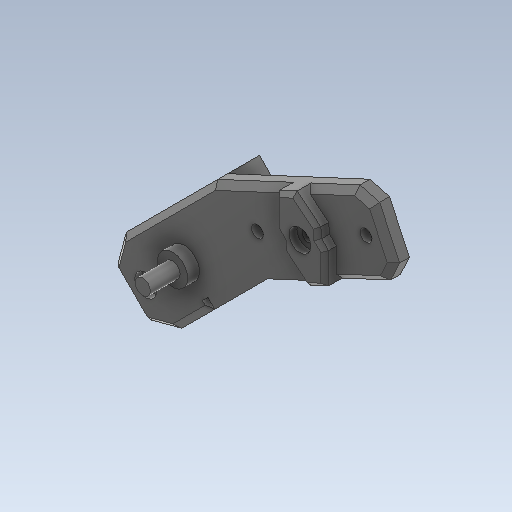
# Autodesk Inventor part: Tibia2Top
Saved by Autodesk Inventor 2020 (Build 240168000, 168)
## iProperties
Created: 2020-09-11
Part Number: Tibia2Top
Material: Generic
Document SubType Name: Modeling
Designer: Turing
Density: 1 g/cm^3
Appearance: Smooth - Black
Mass: 12.5949 g
Surface Area: 55.3576 cm^2
Volume: 12.5949 cm^3
Author: Turing
Autodesk Inventor part; units mm, degrees
ref_plane "YZ Plane" through (0, 0, 0) normal (1, 0, 0) x (0, 1, 0)
ref_plane "XZ Plane" through (0, 0, 0) normal (0, 1, 0) x (-1, 0, 0)
ref_plane "XY Plane" through (0, 0, 0) normal (0, 0, 1) x (1, 0, 0)
sketch "Sketch1" plane through (0, 0, 0) normal (0, 0, 1) x (1, 0, 0)
  circle A0 centre (158.1587, -44.9831) radius 1.5
  circle A1 centre (158.1574, -44.9818) radius 3.6
  line L0 (162.4482, -44.088) -> (170.4914, -34.8578)
  line L1 (167.6018, -32.12) -> (158.8186, -40.6491)
  circle A2 centre (168.8869, -33.6576) radius 1.9999
  line L2 (161.7538, -44.8209) -> (162.4482, -44.088)
  line L3 (158.1242, -41.382) -> (158.8186, -40.6491)
  line L4 (158.1574, -44.9818) -> (168.1574, -44.9818) construction
  line L5 (165.2285, -52.0529) -> (179.3706, -37.9108)
  line L6 (158.1574, -44.9818) -> (168.1574, -44.9818) construction
  line L7 (158.1574, -44.9818) -> (151.0863, -37.9108)
  line L8 (151.0863, -37.9108) -> (165.2285, -23.7686)
  line L9 (165.2285, -23.7686) -> (201.4808, -6.8639)
  line L10 (179.3706, -37.9108) -> (206.5598, -25.2322)
  line L11 (151.0863, -37.9108) -> (141.894, -47.1032)
  line L12 (165.2285, -52.0529) -> (156.0361, -61.2453)
  line L13 (148.3087, -63.3158) -> (156.0361, -61.2453)
  line L14 (141.894, -47.1032) -> (139.8234, -54.8306)
  line L15 (148.3087, -63.3158) -> (139.8234, -54.8306)
  line L16 (209.2788, -23.9644) -> (206.5598, -25.2322)
  line L17 (201.4808, -6.8639) -> (206.4848, -8.2047)
  line L18 (206.4848, -8.2047) -> (211.5562, -19.0804)
  line L19 (211.5562, -19.0804) -> (209.2788, -23.9644)
  point P0 (0, 0)
  point P1 (167.4372, -32.2799)
  point P2 (167.5524, -32.168)
  point P3 (170.4476, -34.9082)
  point P4 (170.3392, -35.0325)
extrude "Extrusion2" add sketch "Sketch1" along normal mid plane 7.5 contours A0 | A1 | A1 L3 L1 A2 L0 L2 | A2 | L12 L13 L15 L14 L11 L8 L9 L17 L18 L19 L16 L10 L5
sketch "Sketch9" plane through (0, 0, 3.75) normal (0, 0, 1) x (1, 0, 0)
  line L0 (156.0361, -61.2453) -> (179.3706, -37.9108) projected
  line L1 (179.3706, -37.9108) -> (209.2788, -23.9644) projected
  line L2 (201.4808, -6.8639) -> (165.2285, -23.7686) projected
  line L3 (165.2285, -23.7686) -> (141.894, -47.1032) projected
  line L4 (141.894, -47.1032) -> (139.8234, -54.8306) projected
  line L5 (139.8234, -54.8306) -> (148.3087, -63.3158) projected
  line L6 (148.3087, -63.3158) -> (156.0361, -61.2453) projected
  line L7 (209.2788, -23.9644) -> (211.5562, -19.0804) projected
  line L8 (211.5562, -19.0804) -> (206.4848, -8.2047) projected
  line L9 (206.4848, -8.2047) -> (201.4808, -6.8639) projected
  point P0 (0, 0)
extrude "Extrusion10" add sketch "Sketch9" along normal blind 5
sketch "Sketch10" plane through (0, 0, 8.75) normal (0, 0, 1) x (1, 0, 0)
  circle A0 centre (158.1587, -44.9831) radius 1.5 projected
  circle A1 centre (158.1587, -44.9831) radius 3.88
  point P0 (0, 0)
  dimension "d155" = 2.38
  constraints: 1 centre point
  measures "d155" radial gap between concentric circles of A0 A1
extrude "Extrusion11" add sketch "Sketch10" along normal blind 3 contours A0 | A1
sketch "Sketch11" plane through (158.1587, -44.9831, 11.75) normal (0, 0, 1) x (1, 0, 0)
  circle A0 centre (0, 0) radius 1.65 projected
  circle A1 centre (0, 0) radius 1.55
  point P0 (-158.1587, 44.9831)
  dimension "d158" = 0.1
  constraints: 1 centre point
  measures "d158" radial gap between concentric circles of A0 A1
extrude "Extrusion12" add sketch "Sketch11" along normal blind 7.6 contours A1
sketch "Sketch15" plane through (0, 0, -3.75) normal (0, 0, -1) x (-1, 0, 0)
  line L0 (-165.2285, -23.7686) -> (-201.4808, -6.8639) projected
  line L1 (-201.4808, -6.8639) -> (-206.4848, -8.2047) projected
  line L2 (-206.4848, -8.2047) -> (-211.5562, -19.0804) projected
  line L3 (-211.5562, -19.0804) -> (-209.2788, -23.9644) projected
  line L4 (-209.2788, -23.9644) -> (-179.3706, -37.9108) projected
  line L5 (-179.3706, -37.9108) -> (-156.0361, -61.2453) projected
  line L6 (-156.0361, -61.2453) -> (-148.3087, -63.3158) projected
  line L7 (-148.3087, -63.3158) -> (-139.8234, -54.8306) projected
  line L8 (-139.8234, -54.8306) -> (-141.894, -47.1032) projected
  line L9 (-141.894, -47.1032) -> (-165.2285, -23.7686) projected
  point P0 (0, 0)
extrude "Extrusion15" cut sketch "Sketch15" against normal blind 0.4
sketch "Sketch25" plane through (0, 0, -3.35) normal (0, 0, -1) x (-1, 0, 0)
  line L0 (-156.0361, -61.2453) -> (-179.3706, -37.9108) projected
  line L1 (-148.3087, -63.3158) -> (-156.0361, -61.2453) projected
  line L2 (-139.8234, -54.8306) -> (-148.3087, -63.3158) projected
  line L3 (-141.894, -47.1032) -> (-139.8234, -54.8306) projected
  line L4 (-165.2285, -23.7686) -> (-141.894, -47.1032) projected
  line L5 (-201.4808, -6.8639) -> (-165.2285, -23.7686) projected
  line L6 (-206.4848, -8.2047) -> (-201.4808, -6.8639) projected
  line L7 (-211.5562, -19.0804) -> (-206.4848, -8.2047) projected
  line L8 (-209.2788, -23.9644) -> (-211.5562, -19.0804) projected
  line L9 (-179.3706, -37.9108) -> (-209.2788, -23.9644) projected
  line L10 (-165.2285, -23.7686) -> (-179.3706, -37.9108)
  point P0 (0, 0)
  constraints: 2 end point
extrude "Extrusion23" cut sketch "Sketch25" against normal blind 8.1 contours L9 L8 L7 L6 L5 L10
sketch "Sketch26" plane through (0, 0, 4.75) normal (0, 0, -1) x (-1, 0, 0)
  line L0 (-201.4808, -6.8639) -> (-165.2285, -23.7686) projected
  line L1 (-206.4848, -8.2047) -> (-201.4808, -6.8639) projected
  line L2 (-211.5562, -19.0804) -> (-206.4848, -8.2047) projected
  line L3 (-209.2788, -23.9644) -> (-211.5562, -19.0804) projected
  line L4 (-179.3706, -37.9108) -> (-209.2788, -23.9644) projected
  line L5 (-165.2285, -23.7686) -> (-179.3706, -37.9108) projected
  line L6 (-209.0205, -13.6426) -> (-172.2995, -30.8397)
  line L7 (-172.2995, -30.8397) -> (-176.8276, -28.7191)
  circle A0 centre (-176.8276, -28.7191) radius 1.55
  line L8 (-209.0205, -13.6426) -> (-204.4924, -15.7631)
  circle A1 centre (-204.4924, -15.7631) radius 1.55
  line L9 (-190.66, -22.2411) -> (-190.6604, -22.242)
  circle A2 centre (-190.6604, -22.242) radius 1.5
  point P0 (0, 0)
  dimension "d262" = 5
  dimension "d263" = 3.1
  dimension "d264" = 5
  dimension "d265" = 3.1
  dimension "d270" = 90
  dimension "d271" = 0.001
  dimension "d272" = 3
  constraints: 8 end point, 3 centre point, 3 coincident, 3 midpoint, 2 point on line
  measures "d262" distance of L6.end L7.end
  measures "d263" diameter of A0
  measures "d264" distance of L6.start L8.end
  measures "d265" diameter of A1
  measures "d270" angle of L6 L9
  measures "d271" distance of L9.start L9.end
  measures "d272" diameter of A2
extrude "Extrusion24" cut sketch "Sketch26" against normal up to surface (4 mm away) contours A0 L6 | L6 A0 | A1 L6 | L6 A1 | A2 L6 | L6 A2
sketch "Sketch27" plane through (0, 0, -3.35) normal (0, 0, -1) x (-1, 0, 0)
  line L0 (-165.2285, -23.7686) -> (-179.3706, -37.9108) projected
  line L1 (-156.0361, -61.2453) -> (-179.3706, -37.9108) projected
  line L2 (-148.3087, -63.3158) -> (-156.0361, -61.2453) projected
  line L3 (-139.8234, -54.8306) -> (-148.3087, -63.3158) projected
  line L4 (-141.894, -47.1032) -> (-139.8234, -54.8306) projected
  line L5 (-165.2285, -23.7686) -> (-141.894, -47.1032) projected
  line L6 (-144.066, -59.0732) -> (-148.3087, -54.8306)
  circle A0 centre (-148.3087, -54.8306) radius 1.5
  point P0 (0, 0)
  dimension "d273" = 6
  dimension "d274" = 90
  dimension "d275" = 3
  constraints: 2 end point, 1 centre point, 1 coincident, 1 midpoint
  measures "d273" distance of L6.start L6.end
  measures "d274" angle of L6 L3
  measures "d275" diameter of A0
extrude "Extrusion25" cut sketch "Sketch27" against normal up to surface (12.1 mm away) contours A0
sketch "Sketch29" plane through (0, 0, 8.75) normal (0, 0, 1) x (1, 0, 0)
  circle A0 centre (148.3087, -54.8306) radius 1.5 projected
  circle A1 centre (204.4924, -15.7631) radius 1.55 projected
  circle A2 centre (190.6604, -22.242) radius 1.5 projected
  circle A3 centre (176.8276, -28.7191) radius 1.55 projected
  circle A4 centre (158.1587, -44.9831) radius 3.88 projected
  line L0 (211.5562, -19.0804) -> (206.4848, -8.2047) projected
  line L1 (206.4848, -8.2047) -> (201.4808, -6.8639) projected
  line L2 (201.4808, -6.8639) -> (165.2285, -23.7686) projected
  line L3 (165.2285, -23.7686) -> (141.894, -47.1032) projected
  line L4 (141.894, -47.1032) -> (139.8234, -54.8306) projected
  line L5 (139.8234, -54.8306) -> (148.3087, -63.3158) projected
  line L6 (148.3087, -63.3158) -> (156.0361, -61.2453) projected
  line L7 (156.0361, -61.2453) -> (179.3706, -37.9108) projected
  line L8 (179.3706, -37.9108) -> (209.2788, -23.9644) projected
  line L9 (209.2788, -23.9644) -> (211.5562, -19.0804) projected
  circle A5 centre (148.3087, -54.8306) radius 2.8
  point P0 (0, 0)
  dimension "d278" = 5.6
  constraints: 1 centre point, 1 coincident
  measures "d278" diameter of A5
extrude "Extrusion26" cut sketch "Sketch29" against normal blind 2 contours A0 | A5
sketch "Sketch30" plane through (0, 0, 8.75) normal (0, 0, 1) x (1, 0, 0)
  circle A0 centre (148.3087, -54.8306) radius 2.8 projected
  circle A1 centre (204.4924, -15.7631) radius 1.55 projected
  circle A2 centre (190.6604, -22.242) radius 1.5 projected
  circle A3 centre (176.8276, -28.7191) radius 1.55 projected
  circle A4 centre (158.1587, -44.9831) radius 3.88 projected
  line L0 (139.8234, -54.8306) -> (148.3087, -63.3158) projected
  line L1 (148.3087, -63.3158) -> (156.0361, -61.2453) projected
  line L2 (156.0361, -61.2453) -> (179.3706, -37.9108) projected
  line L3 (179.3706, -37.9108) -> (209.2788, -23.9644) projected
  line L4 (209.2788, -23.9644) -> (211.5562, -19.0804) projected
  line L5 (211.5562, -19.0804) -> (206.4848, -8.2047) projected
  line L6 (206.4848, -8.2047) -> (201.4808, -6.8639) projected
  line L7 (201.4808, -6.8639) -> (165.2285, -23.7686) projected
  line L8 (165.2285, -23.7686) -> (141.894, -47.1032) projected
  line L9 (141.894, -47.1032) -> (139.8234, -54.8306) projected
  line L10 (190.6604, -22.242) -> (194.6455, -30.788)
  line L11 (190.6604, -22.242) -> (186.7029, -13.755)
  line L12 (190.6604, -22.242) -> (195.192, -20.1289)
  line L13 (190.6604, -22.242) -> (186.1289, -24.3551)
  line L14 (186.1289, -24.3551) -> (184.3611, -22.5874)
  line L15 (186.1289, -24.3551) -> (186.3468, -26.8456)
  line L16 (195.192, -20.1289) -> (194.9741, -17.6385)
  line L17 (195.192, -20.1289) -> (196.9597, -21.8967)
  line L18 (194.6455, -30.788) -> (192.3797, -31.8445)
  line L19 (194.6455, -30.788) -> (196.9112, -29.7314)
  line L20 (186.7029, -13.755) -> (184.4371, -14.8115)
  line L21 (186.7029, -13.755) -> (188.9686, -12.6984)
  line L22 (192.3797, -31.8445) -> (186.3468, -26.8456)
  line L23 (196.9112, -29.7314) -> (196.9597, -21.8967)
  line L24 (194.9741, -17.6385) -> (188.9686, -12.6984)
  line L25 (184.3611, -22.5874) -> (184.4371, -14.8115)
  point P0 (0, 0)
  dimension "d281" = 90
  dimension "d282" = 90
  dimension "d283" = 90
  dimension "d284" = 90
  dimension "d285" = 5
  dimension "d286" = 5
  dimension "d287" = 2.5
  dimension "d288" = 2.5
  dimension "d289" = 2.5
  dimension "d291" = 110
  dimension "d292" = 110
  dimension "d293" = 110
  dimension "d295" = 110
  dimension "d296" = 2.5
  dimension "d297" = 2.5
  dimension "d298" = 2.5
  dimension "d299" = 2.5
  dimension "d300" = 2.5
  constraints: 32 end point, 6 point on line
  measures "d281" angle of L11 L7
  measures "d282" angle of L3 L10
  measures "d283" angle of L10 L13
  measures "d284" angle of L10 L12
  measures "d285" distance of L10.start L13.end
  measures "d286" distance of L10.start L12.end
  measures "d287" distance of L13.end L14.end
  measures "d288" distance of L13.end L15.end
  measures "d289" distance of L12.end L16.end
  measures "d291" angle of L15 L13
  measures "d292" angle of L13 L14
  measures "d293" angle of L16 L12
  measures "d295" angle of L17 L12
  measures "d296" distance of L12.end L17.end
  measures "d297" distance of L10.end L18.end
  measures "d298" distance of L19.end L10.end
  measures "d299" distance of L11.end L20.end
  measures "d300" distance of L11.end L21.end
extrude "Extrusion27" add sketch "Sketch30" along normal blind 3 contours A2 L12 L17 L23 L3 L10 | A2 L11 L7 L24 L16 L12 | L10 L3 L22 L15 L13 A2 | A2 L13 L14 L25 L7 L11
sketch "Sketch31" plane through (0, 0, 11.75) normal (0, 0, 1) x (1, 0, 0)
  line L0 (195.192, -20.1289) -> (194.9741, -17.6385) projected
  line L1 (194.9741, -17.6385) -> (188.9686, -12.6984) projected
  line L2 (188.9686, -12.6984) -> (184.4371, -14.8115) projected
  line L3 (184.4371, -14.8115) -> (184.3611, -22.5874) projected
  line L4 (184.3611, -22.5874) -> (186.1289, -24.3551) projected
  line L5 (186.1289, -24.3551) -> (186.3468, -26.8456) projected
  line L6 (186.3468, -26.8456) -> (192.3797, -31.8445) projected
  line L7 (192.3797, -31.8445) -> (196.9112, -29.7314) projected
  line L8 (196.9112, -29.7314) -> (196.9597, -21.8967) projected
  line L9 (196.9597, -21.8967) -> (195.192, -20.1289) projected
  circle A0 centre (190.6604, -22.242) radius 1.5 projected
  circle A1 centre (190.6604, -22.242) radius 2.8
  point P0 (0, 0)
  dimension "d307" = 5.6
  constraints: 1 centre point, 1 coincident
  measures "d307" diameter of A1
extrude "Extrusion28" cut sketch "Sketch31" against normal blind 2 contours A0 | A1
sketch "Sketch32" plane through (209.2788, -23.9644, 4.75) normal (0.4226183, -0.9063078, 0) x (0.9063078, 0.4226183, 0)
  line L0 (-33, 0) -> (0, 0) projected
  line L1 (0, 0) -> (0, 4) projected
  line L2 (-13.6461, 4) -> (0, 4) projected
  line L3 (-13.6461, 4) -> (-13.6461, 7) projected
  line L4 (-18.6461, 7) -> (-13.6461, 7) projected
  line L5 (-18.6461, 4) -> (-18.6461, 7) projected
  line L6 (-33, 4) -> (-18.6461, 4) projected
  line L7 (-33, 0) -> (-33, 4) projected
  line L8 (-16.1461, 7) -> (-16.1461, 2)
  line L9 (-16.1461, 2) -> (-33, 2)
  line L10 (-16.1461, 2) -> (-15.1461, 2)
  line L11 (-15.1461, 2) -> (-15.1461, 0)
  line L12 (-15.1461, 2) -> (-15.1461, 3)
  line L13 (-16.1461, 2) -> (-17.1461, 2)
  line L14 (-17.1461, 2) -> (-17.1461, 0)
  line L15 (-17.1461, 2) -> (-17.1461, 1)
  line L16 (-17.1461, 1) -> (-33, 1)
  line L17 (-15.1461, 3) -> (-33, 3)
  point P0 (-179.5432, -4.75)
  dimension "d310" = 90
  dimension "d311" = 1
  dimension "d312" = 1
  dimension "d313" = 1
  dimension "d314" = 1
  constraints: 20 end point, 6 point on line, 3 midpoint, 3 perpendicular, 2 vertical, 1 parallel
  measures "d310" angle of L8 L9
  measures "d311" distance of L8.end L10.end
  measures "d312" distance of L10.end L12.end
  measures "d313" distance of L8.end L13.end
  measures "d314" distance of L13.end L15.end
extrude "Extrusion29" cut sketch "Sketch32" against normal blind 2.5 contours L14 L9 L10 L11 L0 | L7 L9 L14 L16 | L7 L17 L8 L9 | L10 L8 L17 L12
sketch "Sketch34" plane through (156.0361, -61.2453, 8.75) normal (0.7071068, -0.7071068, 0) x (-0.7071068, -0.7071068, 0)
  line L0 (0, 12.1) -> (-33, 12.1) projected
  line L1 (-33, 12.1) -> (-33, 4) projected
  line L2 (-33, 4) -> (-33, 3) projected
  line L3 (-33, 3) -> (-33, 1) projected
  line L4 (-33, 1) -> (-33, 0) projected
  line L5 (0, 0) -> (-33, 0) projected
  line L6 (0, 12.1) -> (0, 0) projected
  line L7 (-16.88, -3) -> (-9.12, -3) projected
  line L8 (-9.12, 0) -> (-16.88, 0) projected
  line L9 (-13, 0) -> (-13, 1.5)
  line L10 (-33, 2) -> (-13, 2)
  line L11 (-13, 2) -> (-13, 1.5)
  line L12 (-33, 2) -> (-33, 1)
  line L13 (-33, 1) -> (-14, 1)
  line L14 (-14, 1) -> (-14, 0)
  line L15 (-13, 0) -> (-12, 0)
  line L16 (-12, 0) -> (-12, 3)
  line L17 (-12, 3) -> (-33, 3)
  line L18 (-14.055, 0) -> (-13, 0)
  line L19 (-33, 2) -> (-33, 3)
  point P0 (67.0272, 8.75)
  point P1 (-12, 0)
  point P2 (-14, 0)
  dimension "d323" = 1
  dimension "d324" = 19
  dimension "d325" = 1
  dimension "d326" = 3
  dimension "d327" = 90
  constraints: 22 end point, 5 point on line, 3 perpendicular, 2 collinear, 2 midpoint, 1 horizontal, 1 parallel, 1 vertical
  measures "d323" distance of L10.start L12.end
  measures "d324" distance of L12.end L13.end
  measures "d325" distance of L9.start L15.end
  measures "d326" distance of L15.end L16.end
  measures "d327" angle of L2 L17
extrude "Extrusion31" cut sketch "Sketch34" against normal blind 2.5 contours L17 L16 L5 L9 L11 L10 L3 | L10 L11 L9 L5 L14 L13 L3
sketch "Sketch35" plane through (178.3141, -35.645, 7.75) normal (0.9063078, 0.4226183, 0) x (0, 0, -1)
  line L0 (2, -2.5) -> (2, 0) projected
  line L1 (2, 0) -> (0, 0) projected
  line L2 (0, -2.5) -> (0, 0) projected
  line L3 (2, -2.5) -> (0, -2.5) projected
  point P0 (7.75, 107.6641)
extrude "Extrusion32" cut sketch "Sketch35" against normal blind 1
chamfer "Chamfer20" distance 1 angle 45 10 edges at (196.9355, -25.8141, 11.75) (196.0759, -21.0128, 11.75) (195.083, -18.8837, 11.75) (191.9714, -15.1684, 11.75) (186.7029, -13.755, 11.75) (184.3991, -18.6994, 11.75) (185.245, -23.4712, 11.75) (186.2378, -25.6004, 11.75) (189.3632, -29.3451, 11.75) (194.6455, -30.788, 11.75)
chamfer "Chamfer22" distance 1.5 angle 45 11 edges at (160.2787, -57.0026, 8.75) (152.1724, -62.2806, 8.75) (144.066, -59.0732, 8.75) (140.8587, -50.9669, 8.75) (153.5612, -35.4359, 8.75) (174.8328, -19.2901, 8.75) (195.2247, -9.7812, 8.75) (203.9828, -7.5343, 8.75) (209.0205, -13.6426, 8.75) (210.4175, -21.5224, 8.75) (203.095, -26.8479, 8.75)
sketch "Sketch37" plane through (158.1587, -44.9831, 19.35) normal (0, 0, 1) x (1, 0, 0)
  circle A0 centre (0, 0) radius 1.55 projected
  circle A1 centre (0, 0) radius 1.95
  point P0 (-158.1587, 44.9831)
  dimension "d353" = 3.9
  constraints: 1 centre point, 1 coincident
  measures "d353" diameter of A1
extrude "Extrusion34" add sketch "Sketch37" against normal blind 7.6
body "Solid2"
